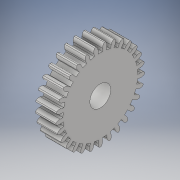
# Autodesk Inventor part: wheel gear
Saved by Autodesk Inventor 2018 (Build 220112000, 112)
## iProperties
Created: 2017-12-18
Part Number: wheel gear
Material: Generic
Document SubType Name: Modeling
Designer: kcmat
Density: 1 g/cm^3
Appearance: Default
Author: kcmat
Autodesk Inventor part; units mm, degrees
ref_plane "YZ Plane" through (0, 0, 0) normal (1, 0, 0) x (0, 1, 0)
ref_plane "XZ Plane" through (0, 0, 0) normal (0, 1, 0) x (-1, 0, 0)
ref_plane "XY Plane" through (0, 0, 0) normal (0, 0, 1) x (1, 0, 0)
sketch "Sketch1" plane through (0, 0, 0) normal (1, 0, 0) x (0, 1, 0)
  circle A0 centre (0, 0) radius 12.7
  line L0 (-12.6663, -1.1327) -> (-12.6581, -1.1327) construction
  arc A1 (-15.0895, 0.2429) -> (-15.0895, -0.246) centre (9.5118, -0.0016) ccw
  line L1 (-13.6508, -0.7286) -> (-12.6913, -0.6565)
  line L2 (-13.6508, 0.7254) -> (-12.6913, 0.6534)
  line L3 (-12.6913, -0.6565) -> (-12.6831, -0.6558)
  line L4 (-12.6913, 0.6534) -> (-12.6832, 0.6526)
  arc A2 (-12.6832, 0.6526) -> (-12.6831, -0.6558) centre (0, 0) ccw
  circle A3 centre (0, 0) radius 2.4892
  arc A4 (-15.0895, -0.246) -> (-13.6508, -0.7286) centre (-13.8463, 1.0744) ccw
  arc A5 (-13.6508, 0.7254) -> (-15.0895, 0.2429) centre (-13.8865, -0.9578) ccw
  line L5 (-12.1267, -3.8292) -> (-12.1186, -3.8274) construction
  arc A6 (-14.7889, -3.0065) -> (-14.6838, -3.4841) centre (9.2898, 2.0432) ccw
  line L6 (-13.175, -3.646) -> (-12.2535, -3.3694)
  line L7 (-13.4876, -2.226) -> (-12.5351, -2.0902)
  line L8 (-12.2535, -3.3694) -> (-12.2455, -3.367)
  line L9 (-12.5351, -2.0902) -> (-12.527, -2.0892)
  arc A7 (-12.527, -2.0892) -> (-12.2455, -3.367) centre (0, 0) ccw
  arc A8 (-14.6838, -3.4841) -> (-13.175, -3.646) centre (-13.7536, -1.9272) ccw
  arc A9 (-13.4876, -2.226) -> (-14.7889, -3.0065) centre (-13.3559, -3.9206) ccw
  line L10 (-11.02, -6.3465) -> (-11.0125, -6.343) construction
  arc A10 (-13.7968, -6.1154) -> (-13.5915, -6.5592) centre (8.6333, 3.9925) ccw
  line L11 (-12.0832, -6.393) -> (-11.2427, -5.9247)
  line L12 (-12.6937, -5.0734) -> (-11.7927, -4.736)
  line L13 (-11.2427, -5.9247) -> (-11.2354, -5.9207)
  line L14 (-11.7927, -4.736) -> (-11.785, -4.7333)
  arc A11 (-11.785, -4.7333) -> (-11.2354, -5.9207) centre (0, 0) ccw
  arc A12 (-13.5915, -6.5592) -> (-12.0832, -6.393) centre (-13.0177, -4.8388) ccw
  arc A13 (-12.6937, -5.0734) -> (-13.7968, -6.1154) centre (-12.2009, -6.7) ccw
  line L15 (-9.3981, -8.5671) -> (-9.3915, -8.5621) construction
  arc A14 (-12.1596, -8.9384) -> (-11.8637, -9.3276) centre (7.5732, 5.7551) ccw
  line L16 (-10.4264, -8.8411) -> (-9.7062, -8.2031)
  line L17 (-11.3063, -7.6836) -> (-10.4989, -7.1603)
  line L18 (-9.7062, -8.2031) -> (-9.7, -8.1976)
  line L19 (-10.4989, -7.1603) -> (-10.492, -7.156)
  arc A15 (-10.492, -7.156) -> (-9.7, -8.1976) centre (0, 0) ccw
  arc A16 (-11.8637, -9.3276) -> (-10.4264, -8.8411) centre (-11.6732, -7.5241) ccw
  arc A17 (-11.3063, -7.6836) -> (-12.1596, -8.9384) centre (-10.4753, -9.1662) ccw
  line L20 (-7.3367, -10.3871) -> (-7.3313, -10.3808) construction
  arc A18 (-9.9539, -11.3433) -> (-9.5812, -11.6599) centre (6.159, 7.2485) ccw
  line L21 (-8.282, -10.8758) -> (-7.7159, -10.0978)
  line L22 (-9.3902, -9.9345) -> (-8.7141, -9.2499)
  line L23 (-7.7159, -10.0978) -> (-7.711, -10.0911)
  line L24 (-8.7141, -9.2499) -> (-8.7083, -9.2442)
  arc A19 (-8.7083, -9.2442) -> (-7.711, -10.0911) centre (0, 0) ccw
  arc A20 (-9.5812, -11.6599) -> (-8.282, -10.8758) centre (-9.7828, -9.8576) ccw
  arc A21 (-9.3902, -9.9345) -> (-9.9539, -11.3433) centre (-8.2599, -11.2038) ccw
  line L25 (-4.9322, -11.7214) -> (-4.9284, -11.7142) construction
  arc A22 (-7.2827, -13.2179) -> (-6.8507, -13.447) centre (4.4568, 8.4031) ccw
  line L26 (-5.7504, -12.4019) -> (-5.3647, -11.5204)
  line L27 (-7.0351, -11.7208) -> (-6.522, -10.9069)
  line L28 (-5.3647, -11.5204) -> (-5.3614, -11.5128)
  line L29 (-6.522, -10.9069) -> (-6.5175, -10.9001)
  arc A23 (-6.5175, -10.9001) -> (-5.3614, -11.5128) centre (0, 0) ccw
  arc A24 (-6.8507, -13.447) -> (-5.7504, -12.4019) centre (-7.435, -11.7301) ccw
  arc A25 (-7.0351, -11.7208) -> (-7.2827, -13.2179) centre (-5.6583, -12.7175) ccw
  line L30 (-2.2971, -12.5077) -> (-2.2949, -12.4997) construction
  arc A26 (-4.2709, -14.4745) -> (-3.7998, -14.6053) centre (2.5462, 9.1647) ccw
  line L31 (-2.95, -13.3481) -> (-2.7627, -12.4043)
  line L32 (-4.351, -12.9591) -> (-4.0248, -12.0539)
  line L33 (-2.7627, -12.4043) -> (-2.7611, -12.3962)
  line L34 (-4.0248, -12.0539) -> (-4.0219, -12.0463)
  arc A27 (-4.0219, -12.0463) -> (-2.7611, -12.3962) centre (0, 0) ccw
  arc A28 (-3.7998, -14.6053) -> (-2.95, -13.3481) centre (-4.7396, -13.0542) ccw
  arc A29 (-4.351, -12.9591) -> (-4.2709, -14.4745) centre (-2.7922, -13.6366) ccw
  line L35 (0.4453, -12.7091) -> (0.4458, -12.7008) construction
  arc A30 (-1.0595, -15.0542) -> (-0.5712, -15.0806) centre (0.5165, 9.4978) ccw
  line L36 (-0.0115, -13.6702) -> (-0.0316, -12.7083)
  line L37 (-1.4634, -13.5915) -> (-1.3395, -12.6373)
  line L38 (-0.0316, -12.7083) -> (-0.0318, -12.7)
  line L39 (-1.3395, -12.6373) -> (-1.3383, -12.6293)
  arc A31 (-1.3383, -12.6293) -> (-0.0318, -12.7) centre (0, 0) ccw
  arc A32 (-0.5712, -15.0806) -> (-0.0115, -13.6702) centre (-1.8225, -13.7678) ccw
  arc A33 (-1.4634, -13.5915) -> (-1.0595, -15.0542) centre (0.2046, -13.918) ccw
  line L40 (3.167, -12.3162) -> (3.1657, -12.3081) construction
  arc A34 (2.2015, -14.93) -> (2.684, -14.8509) centre (-1.5373, 9.3867) ccw
  line L41 (2.9274, -13.3531) -> (2.701, -12.4179)
  line L42 (1.4926, -13.5883) -> (1.4085, -12.6298)
  line L43 (2.701, -12.4179) -> (2.6991, -12.4099)
  line L44 (1.4085, -12.6298) -> (1.4079, -12.6217)
  arc A35 (1.4079, -12.6217) -> (2.6991, -12.4099) centre (0, 0) ccw
  arc A36 (2.684, -14.8509) -> (2.9274, -13.3531) centre (1.1798, -13.8377) ccw
  arc A37 (1.4926, -13.5883) -> (2.2015, -14.93) centre (3.1917, -13.5486) ccw
  line L45 (5.7406, -11.3475) -> (5.7375, -11.3398) construction
  arc A38 (5.3595, -14.1077) -> (5.8137, -13.9267) centre (-3.5192, 8.8368) ccw
  line L46 (5.7295, -12.4116) -> (5.3074, -11.547)
  line L47 (4.3788, -12.9498) -> (4.0906, -12.0318)
  line L48 (5.3074, -11.547) -> (5.3038, -11.5395)
  line L49 (4.0906, -12.0318) -> (4.0883, -12.024)
  arc A39 (4.0883, -12.024) -> (5.3038, -11.5395) centre (0, 0) ccw
  arc A40 (5.8137, -13.9267) -> (5.7295, -12.4116) centre (4.1269, -13.2606) ccw
  arc A41 (4.3788, -12.9498) -> (5.3595, -14.1077) centre (6.0297, -12.5457) ccw
  line L50 (8.0457, -9.8481) -> (8.0411, -9.8413) construction
  arc A42 (8.2669, -12.6257) -> (8.6717, -12.3513) centre (-5.3366, 7.8737) ccw
  line L51 (8.2637, -10.8897) -> (7.6656, -10.1361)
  line L52 (7.0602, -11.7057) -> (6.5814, -10.8711)
  line L53 (7.6656, -10.1361) -> (7.6604, -10.1296)
  line L54 (6.5814, -10.8711) -> (6.5775, -10.864)
  arc A43 (6.5775, -10.864) -> (7.6604, -10.1296) centre (0, 0) ccw
  arc A44 (8.6717, -12.3513) -> (8.2637, -10.8897) centre (6.8811, -12.0634) ccw
  arc A45 (7.0602, -11.7057) -> (8.2669, -12.6257) centre (8.5857, -10.9562) ccw
  line L55 (9.9747, -7.8883) -> (9.9687, -7.8826) construction
  arc A46 (10.7878, -10.5534) -> (11.1241, -10.1984) centre (-6.9044, 6.5424) ccw
  line L56 (10.4114, -8.8587) -> (9.6653, -8.2512)
  line L57 (9.4115, -9.9143) -> (8.7645, -9.2021)
  line L58 (9.6653, -8.2512) -> (9.6589, -8.246)
  line L59 (8.7645, -9.2021) -> (8.7592, -9.196)
  arc A47 (8.7592, -9.196) -> (9.6589, -8.246) centre (0, 0) ccw
  arc A48 (11.1241, -10.1984) -> (10.4114, -8.8587) centre (9.3135, -10.3021) ccw
  arc A49 (9.4115, -9.9143) -> (10.7878, -10.5534) centre (10.7402, -8.8544) ccw
  line L60 (11.4372, -5.5596) -> (11.4302, -5.5553) construction
  arc A50 (12.8043, -7.9876) -> (13.0564, -7.5686) centre (-8.1494, 4.9052) ccw
  line L61 (12.0724, -6.4134) -> (11.2131, -5.9806)
  line L62 (11.3228, -7.6593) -> (10.5378, -7.1029)
  line L63 (11.2131, -5.9806) -> (11.2057, -5.9768)
  line L64 (10.5378, -7.1029) -> (10.5313, -7.0981)
  arc A51 (10.5313, -7.0981) -> (11.2057, -5.9768) centre (0, 0) ccw
  arc A52 (13.0564, -7.5686) -> (12.0724, -6.4134) centre (11.3104, -8.0592) ccw
  arc A53 (11.3228, -7.6593) -> (12.8043, -7.9876) centre (12.3925, -6.3386) ccw
  line L65 (12.365, -2.9709) -> (12.3572, -2.9683) construction
  arc A54 (14.222, -5.0483) -> (14.3781, -4.5849) centre (-9.0134, 3.0386) ccw
  line L66 (13.1688, -3.6683) -> (12.2366, -3.4303)
  line L67 (12.7046, -5.0462) -> (11.8184, -4.6715)
  line L68 (12.2366, -3.4303) -> (12.2286, -3.4282)
  line L69 (11.8184, -4.6715) -> (11.8109, -4.6682)
  arc A55 (11.8109, -4.6682) -> (12.2286, -3.4282) centre (0, 0) ccw
  arc A56 (14.3781, -4.5849) -> (13.1688, -3.6683) centre (12.7784, -5.4394) ccw
  arc A57 (12.7046, -5.0462) -> (14.222, -5.0483) centre (13.4654, -3.5263) ccw
  line L70 (12.7146, -0.2434) -> (12.7064, -0.2425) construction
  arc A58 (14.9747, -1.873) -> (15.0276, -1.3869) centre (-9.4559, 1.03) ccw
  line L71 (13.6495, -0.7516) -> (12.6879, -0.7196)
  line L72 (13.4923, -2.1971) -> (12.5463, -2.0217)
  line L73 (12.6879, -0.7196) -> (12.6796, -0.7193)
  line L74 (12.5463, -2.0217) -> (12.5383, -2.0201)
  arc A59 (12.5383, -2.0201) -> (12.6796, -0.7193) centre (0, 0) ccw
  arc A60 (15.0276, -1.3869) -> (13.6495, -0.7516) centre (13.649, -2.5652) ccw
  arc A61 (13.4923, -2.1971) -> (14.9747, -1.873) centre (13.9086, -0.5492) ccw
  line L75 (12.4696, 2.4956) -> (12.4614, 2.4947) construction
  arc A62 (15.0273, 1.39) -> (14.9744, 1.8761) centre (-9.4562, -1.0269) ccw
  line L76 (13.492, 2.2002) -> (12.5459, 2.0248)
  line L77 (13.6492, 0.7547) -> (12.6876, 0.7227)
  line L78 (12.5459, 2.0248) -> (12.5378, 2.0233)
  line L79 (12.6876, 0.7227) -> (12.6794, 0.7225)
  arc A63 (12.6794, 0.7225) -> (12.5378, 2.0233) centre (0, 0) ccw
  arc A64 (14.9744, 1.8761) -> (13.492, 2.2002) centre (13.8813, 0.4289) ccw
  arc A65 (13.6492, 0.7547) -> (15.0273, 1.39) centre (13.7015, 2.4536) ccw
  line L80 (11.6416, 5.1178) -> (11.6338, 5.1152) construction
  arc A66 (14.3771, 4.5879) -> (14.221, 5.0512) centre (-9.0144, -3.0357) ccw
  line L81 (12.7036, 5.0491) -> (11.8174, 4.6745)
  line L82 (13.1678, 3.6712) -> (12.2356, 3.4332)
  line L83 (11.8174, 4.6745) -> (11.8097, 4.6712)
  line L84 (12.2356, 3.4332) -> (12.2277, 3.4313)
  arc A67 (12.2277, 3.4313) -> (11.8097, 4.6712) centre (0, 0) ccw
  arc A68 (14.221, 5.0512) -> (12.7036, 5.0491) centre (13.4646, 3.4029) ccw
  arc A69 (13.1678, 3.6712) -> (14.3771, 4.5879) centre (12.8538, 5.3416) ccw
  line L85 (10.2692, 7.5008) -> (10.2622, 7.4965) construction
  arc A70 (13.0547, 7.5713) -> (12.8027, 7.9902) centre (-8.1511, -4.9025) ccw
  line L86 (11.3212, 7.662) -> (10.5362, 7.1056)
  line L87 (12.0708, 6.4161) -> (11.2115, 5.9832)
  line L88 (10.5362, 7.1056) -> (10.5294, 7.1008)
  line L89 (11.2115, 5.9832) -> (11.2042, 5.9797)
  arc A71 (11.2042, 5.9797) -> (10.5294, 7.1008) centre (0, 0) ccw
  arc A72 (12.8027, 7.9902) -> (11.3212, 7.662) centre (12.4182, 6.2179) ccw
  arc A73 (12.0708, 6.4161) -> (13.0547, 7.5713) centre (11.405, 7.9799) ccw
  line L90 (8.4167, 9.533) -> (8.4107, 9.5273) construction
  arc A74 (11.1219, 10.2007) -> (10.7857, 10.5556) centre (-6.9066, -6.5401) ccw
  line L91 (9.4094, 9.9166) -> (8.7624, 9.2044)
  line L92 (10.4093, 8.861) -> (9.6632, 8.2535)
  line L93 (8.7624, 9.2044) -> (8.7568, 9.1983)
  line L94 (9.6632, 8.2535) -> (9.6567, 8.2485)
  arc A75 (9.6567, 8.2485) -> (8.7568, 9.1983) centre (0, 0) ccw
  arc A76 (10.7857, 10.5556) -> (9.4094, 9.9166) centre (10.7913, 8.7421) ccw
  arc A77 (10.4093, 8.861) -> (11.1219, 10.2007) centre (9.4229, 10.2451) ccw
  line L95 (6.1706, 11.1195) -> (6.166, 11.1126) construction
  arc A78 (8.6691, 12.3531) -> (8.2644, 12.6275) centre (-5.3392, -7.8719) ccw
  line L96 (7.0576, 11.7075) -> (6.5789, 10.8729)
  line L97 (8.2611, 10.8915) -> (7.663, 10.1378)
  line L98 (6.5789, 10.8729) -> (6.5747, 10.8657)
  line L99 (7.663, 10.1378) -> (7.6578, 10.1315)
  arc A79 (7.6578, 10.1315) -> (6.5747, 10.8657) centre (0, 0) ccw
  arc A80 (8.2644, 12.6275) -> (7.0576, 11.7075) centre (8.6597, 10.8575) ccw
  arc A81 (8.2611, 10.8915) -> (8.6691, 12.3531) centre (7.0002, 12.0312) ccw
  line L100 (3.636, 12.186) -> (3.6329, 12.1783) construction
  arc A82 (5.8109, 13.9278) -> (5.3566, 14.1088) centre (-3.5221, -8.8357) ccw
  line L101 (4.3759, 12.9509) -> (4.0877, 12.0329)
  line L102 (5.7266, 12.4127) -> (5.3045, 11.5481)
  line L103 (4.0877, 12.0329) -> (4.0852, 12.025)
  line L104 (5.3045, 11.5481) -> (5.3008, 11.5409)
  arc A83 (5.3008, 11.5409) -> (4.0852, 12.025) centre (0, 0) ccw
  arc A84 (5.3566, 14.1088) -> (4.3759, 12.9509) centre (6.1232, 12.4652) ccw
  arc A85 (5.7266, 12.4127) -> (5.8109, 13.9278) centre (4.2502, 13.2547) ccw
  line L105 (0.9314, 12.6827) -> (0.93, 12.6746) construction
  arc A86 (2.6809, 14.8514) -> (2.1984, 14.9305) centre (-1.5404, -9.3862) ccw
  line L106 (1.4895, 13.5888) -> (1.4054, 12.6303)
  line L107 (2.9243, 13.3536) -> (2.698, 12.4184)
  line L108 (1.4054, 12.6303) -> (1.4047, 12.6221)
  line L109 (2.698, 12.4184) -> (2.6959, 12.4106)
  arc A87 (2.6959, 12.4106) -> (1.4047, 12.6221) centre (0, 0) ccw
  arc A88 (2.1984, 14.9305) -> (1.4895, 13.5888) centre (3.3004, 13.4901) ccw
  arc A89 (2.9243, 13.3536) -> (2.6809, 14.8514) centre (1.3014, 13.8585) ccw
  line L110 (-1.8168, 12.5864) -> (-1.8164, 12.5782) construction
  arc A90 (-0.5744, 15.0805) -> (-1.0626, 15.054) centre (0.5134, -9.4979) ccw
  line L111 (-1.4665, 13.5913) -> (-1.3426, 12.6372)
  line L112 (-0.0147, 13.67) -> (-0.0347, 12.7081)
  line L113 (-1.3426, 12.6372) -> (-1.3415, 12.6289)
  line L114 (-0.0347, 12.7081) -> (-0.035, 12.7)
  arc A91 (-0.035, 12.7) -> (-1.3415, 12.6289) centre (0, 0) ccw
  arc A92 (-1.0626, 15.054) -> (-1.4665, 13.5913) centre (0.3232, 13.8842) ccw
  arc A93 (-0.0147, 13.67) -> (-0.5744, 15.0805) centre (-1.7082, 13.8143) ccw
  line L115 (-4.4801, 11.9016) -> (-4.4779, 11.8937) construction
  arc A94 (-3.8028, 14.6044) -> (-4.2739, 14.4736) centre (2.5432, -9.1655) ccw
  line L116 (-4.354, 12.9583) -> (-4.0278, 12.0531)
  line L117 (-2.953, 13.3473) -> (-2.7658, 12.4035)
  line L118 (-4.0278, 12.0531) -> (-4.025, 12.0453)
  line L119 (-2.7658, 12.4035) -> (-2.7643, 12.3955)
  arc A95 (-2.7643, 12.3955) -> (-4.025, 12.0453) centre (0, 0) ccw
  arc A96 (-4.2739, 14.4736) -> (-4.354, 12.9583) centre (-2.669, 13.6291) ccw
  arc A97 (-2.953, 13.3473) -> (-3.8028, 14.6044) centre (-4.6379, 13.1241) ccw
  line L120 (-6.9338, 10.6603) -> (-6.93, 10.653) construction
  arc A98 (-6.8534, 13.4455) -> (-7.2854, 13.2165) centre (4.454, -8.4045) ccw
  line L121 (-7.0378, 11.7194) -> (-6.5247, 10.9054)
  line L122 (-5.7532, 12.4004) -> (-5.3675, 11.519)
  line L123 (-6.5247, 10.9054) -> (-6.5203, 10.8984)
  line L124 (-5.3675, 11.519) -> (-5.3644, 11.5115)
  arc A99 (-5.3644, 11.5115) -> (-6.5203, 10.8984) centre (0, 0) ccw
  arc A100 (-7.2854, 13.2165) -> (-7.0378, 11.7194) centre (-5.5364, 12.7367) ccw
  arc A101 (-5.7532, 12.4004) -> (-6.8534, 13.4455) centre (-7.3508, 11.8203) ccw
  line L125 (-9.0633, 8.9205) -> (-9.058, 8.9142) construction
  arc A102 (-9.5836, 11.6579) -> (-9.9562, 11.3413) centre (6.1566, -7.2505) ccw
  line L126 (-9.3926, 9.9324) -> (-8.7165, 9.2479)
  line L127 (-8.2844, 10.8738) -> (-7.7182, 10.0958)
  line L128 (-8.7165, 9.2479) -> (-8.7107, 9.242)
  line L129 (-7.7182, 10.0958) -> (-7.7136, 10.0891)
  arc A103 (-7.7136, 10.0891) -> (-8.7107, 9.242) centre (0, 0) ccw
  arc A104 (-9.9562, 11.3413) -> (-9.3926, 9.9324) centre (-8.145, 11.2487) ccw
  arc A105 (-8.2844, 10.8738) -> (-9.5836, 11.6579) centre (-9.7199, 9.9637) ccw
  line L130 (-10.7691, 6.7636) -> (-10.7625, 6.7586) construction
  arc A106 (-11.8656, 9.3251) -> (-12.1615, 8.9359) centre (7.5713, -5.7575) ccw
  line L131 (-11.3082, 7.6811) -> (-10.5008, 7.1578)
  line L132 (-10.4283, 8.8386) -> (-9.7081, 8.2006)
  line L133 (-10.5008, 7.1578) -> (-10.4938, 7.1533)
  line L134 (-9.7081, 8.2006) -> (-9.7021, 8.1951)
  arc A107 (-9.7021, 8.1951) -> (-10.4938, 7.1533) centre (0, 0) ccw
  arc A108 (-12.1615, 8.9359) -> (-11.3082, 7.6811) centre (-10.3727, 9.2348) ccw
  arc A109 (-10.4283, 8.8386) -> (-11.8656, 9.3251) centre (-11.6346, 7.6413) ccw
  line L135 (-11.9713, 4.2904) -> (-11.9638, 4.2869) construction
  arc A110 (-13.5928, 6.5564) -> (-13.7981, 6.1126) centre (8.632, -3.9953) ccw
  line L136 (-12.695, 5.0706) -> (-11.794, 4.7332)
  line L137 (-12.0845, 6.3902) -> (-11.244, 5.9219)
  line L138 (-11.794, 4.7332) -> (-11.7862, 4.7302)
  line L139 (-11.244, 5.9219) -> (-11.237, 5.9178)
  arc A111 (-11.237, 5.9178) -> (-11.7862, 4.7302) centre (0, 0) ccw
  arc A112 (-13.7981, 6.1126) -> (-12.695, 5.0706) centre (-12.1154, 6.7891) ccw
  arc A113 (-12.0845, 6.3902) -> (-13.5928, 6.5564) centre (-13.0052, 4.9615) ccw
  line L140 (-12.6137, 1.6166) -> (-12.6057, 1.6149) construction
  arc A114 (-14.6845, 3.481) -> (-14.7896, 3.0035) centre (9.2891, -2.0463) ccw
  line L141 (-13.4883, 2.223) -> (-12.5357, 2.0871)
  line L142 (-13.1757, 3.643) -> (-12.2542, 3.3663)
  line L143 (-12.5357, 2.0871) -> (-12.5275, 2.086)
  line L144 (-12.2542, 3.3663) -> (-12.2464, 3.3639)
  arc A115 (-12.2464, 3.3639) -> (-12.5275, 2.086) centre (0, 0) ccw
  arc A116 (-14.7896, 3.0035) -> (-13.4883, 2.223) centre (-13.2916, 4.0259) ccw
  arc A117 (-13.1757, 3.643) -> (-14.6845, 3.481) centre (-13.7677, 2.0498) ccw
  dimension "d0" = 25.4
  dimension "d16" = 4.9784
  dimension "d37" = 360
  constraints: 290 end point, 234 point on circle, 118 centre point, 1 coincident, 1 concentric, 1 horizontal, 668 other
  measures "d0" diameter of A0
  measures "d16" diameter of A3
extrude "Extrusion6" add sketch "Sketch1" along normal blind 7
sketch "Sketch2" plane through (0, 0, 0) normal (-1, 0, 0) x (0, 0, 1)
  circle A0 centre (0, 0) radius 3.175
  dimension "d41" = 6.35
  constraints: 1 centre point, 1 coincident
  measures "d41" diameter of A0
extrude "Extrusion7" cut sketch "Sketch2" against normal blind 7
sketch "Sketch3" plane through (7, 0, 0) normal (1, 0, 0) x (0, 0, -1)
  circle A0 centre (0, 0) radius 3.175 projected
  circle A1 centre (0, 0) radius 3.556
  dimension "d44" = 7.112
  constraints: 1 centre point, 1 coincident
  measures "d44" diameter of A1
extrude "Extrusion8" cut sketch "Sketch3" against normal blind 10
body "Solid6"
